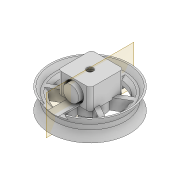
# Autodesk Inventor part: Primary_hinge
Saved by Autodesk Inventor 2022 (Build 260153000, 153)
## iProperties
Created: 2022-07-14
Part Number: Primary_hinge
Material: Generic
Document SubType Name: Modeling
Designer: dell
Density: 1 g/cm^3
Appearance: Default
Mass: 10.1293 g
Surface Area: 99.4908 cm^2
Volume: 10.1293 cm^3
Author: dell
Autodesk Inventor part; units mm, degrees
ref_plane "XZ Plane" through (0, 0, 0) normal (0, 1, 0) x (-1, 0, 0)
ref_plane "XY Plane" through (0, 0, 0) normal (0, 0, 1) x (1, 0, 0)
sketch "Sketch1" plane through (0, 0, 0) normal (0, 0, 1) x (1, 0, 0)
  circle A0 centre (0, 0) radius 4.9
  circle A1 centre (0, 0) radius 6.1
  line L0 (-10.1, -7.1) -> (10.1, -7.1)
  line L1 (10.1, -7.1) -> (10.1, 7.1)
  line L2 (10.1, 7.1) -> (-10.1, 7.1)
  line L3 (-10.1, 7.1) -> (-10.1, -7.1)
  line L4 (-10.1, -7.1) -> (10.1, 7.1) construction
  line L5 (10.1, -7.1) -> (-10.1, 7.1) construction
  dimension "d0" = 9.8
  dimension "d1" = 12.2
  dimension "d3" = 4
  dimension "d4" = 1
  constraints: 12 end point, 2 centre point, 2 coincident, 2 midpoint, 2 parallel, 1 horizontal, 1 perpendicular
  measures "d0" diameter of A0
  measures "d1" diameter of A1
  measures "d3" distance edge to line of A1 L1
  measures "d4" distance edge to line of A1 L2
extrude "Extrusion1" add sketch "Sketch1" along normal blind 18
sketch "Sketch2" plane through (0, 0, 18) normal (0, 0, 1) x (1, 0, 0)
  circle A0 centre (0, 0) radius 4.9 projected
extrude "Extrusion2" add sketch "Sketch2" along normal blind 2
sketch "Sketch3" plane through (0, 0, 0) normal (0, 0, -1) x (-1, 0, 0)
  line L0 (-10.1, -7.1) -> (-10.1, 7.1) projected
  line L1 (10.1, -7.1) -> (-10.1, -7.1) projected
  line L2 (10.1, 7.1) -> (10.1, -7.1) projected
  line L3 (-10.1, 7.1) -> (10.1, 7.1) projected
  circle A0 centre (0, 0) radius 6.1 projected
extrude "Extrusion3" add sketch "Sketch3" along normal blind 3 contours L0 L3 L2 L1 | A0
ref_plane "Work Plane1" through (0, -7.1, 18) normal (-1, 0, 0) x (0, 0, 1)
sketch "Sketch6" plane through (-10.1, 7.1, 18) normal (0, 1, 0) x (1, 0, 0)
  line L0 (5.2, 18) -> (15, 18) projected
  line L1 (16.2, 18) -> (4, 18) projected
  line L2 (20.2, 0) -> (0, 0) projected
  line L3 (0, 21) -> (20.2, 21) projected
  line L4 (16.2, 0) -> (16.2, 18) projected
  line L5 (4, 0) -> (4, 18) projected
  circle A0 centre (10.1, 10) radius 2.05
  line L6 (0, 21) -> (0, 0) projected
  line L7 (20.2, 21) -> (20.2, 0) projected
  point P0 (10.1, 18)
  point P1 (10.1, 18)
  dimension "d49" = 4.1
  dimension "d50" = 10
  constraints: 1 centre point, 1 coincident, 1 midpoint, 1 vertical alignment
  measures "d49" diameter of A0
  measures "d50" distance from line of L2 A0.centre
extrude "Extrusion12" cut sketch "Sketch6" against normal blind 100 contours A0
fillet "Fillet5" radius 2 4 edges at (10.1, 0, 18) (-10.1, 0, 18) (10.1, 0, -3) (-10.1, 0, -3)
sketch "Sketch14" plane through (-8.1, -7.1, -3) normal (0, -1, 0) x (1, 0, 0)
  circle A0 centre (8.1, 11) radius 2.05
  line L0 (8.1, 15.041452) -> (11.6, 13.020726)
  line L1 (11.6, 13.020726) -> (11.6, 8.979274)
  line L2 (11.6, 8.979274) -> (8.1, 6.958548)
  line L3 (8.1, 6.958548) -> (4.6, 8.979274)
  line L4 (4.6, 8.979274) -> (4.6, 13.020726)
  line L5 (4.6, 13.020726) -> (8.1, 15.041452)
  circle A1 centre (8.1, 11) radius 8
  point P0 (8.1, 3)
  dimension "d69" = 7
  dimension "d73" = 16
  constraints: 12 end point, 2 coincident, 1 centre point, 13 other
  measures "d69" distance between parallel lines of L1 L4
  measures "d73" diameter of A1
extrude "Extrusion14" add sketch "Sketch14" along normal blind 5 contours A1
sketch "Sketch15" plane through (0, -12.1, 8) normal (0, -1, 0) x (1, 0, 0)
  line L0 (3.4, -1) -> (4.8, -1)
  line L1 (4.8, -1) -> (4.8, -7.241547)
  line L2 (4.8, -7.241547) -> (3.4, -7.241547)
  line L3 (3.4, -7.241547) -> (3.4, -1)
  line L4 (3.4, -1) -> (4.8, -7.241547) construction
  line L5 (4.8, -1) -> (3.4, -7.241547) construction
  line L6 (0, 16.6) -> (0, -15.6)
  circle A0 centre (0, 0) radius 2.05
  circle A1 centre (0, 0) radius 4.5
  circle A2 centre (0, 0) radius 8
  line L7 (0, 4.041452) -> (3.5, 2.020726)
  line L8 (3.5, 2.020726) -> (3.5, -2.020726)
  line L9 (3.5, -2.020726) -> (0, -4.041452)
  line L10 (0, -4.041452) -> (-3.5, -2.020726)
  line L11 (-3.5, -2.020726) -> (-3.5, 2.020726)
  line L12 (-3.5, 2.020726) -> (0, 4.041452)
  circle A3 centre (0, 0) radius 8
  line L13 (1.4, -7.876547) -> (3.4, -7.876547)
  line L14 (3.4, -7.876547) -> (3.4, -4.876547)
  line L15 (3.4, -4.876547) -> (1.4, -4.876547)
  line L16 (1.4, -4.876547) -> (1.4, -7.876547)
  line L17 (4.8, -6.4) -> (6.8, -6.4)
  line L18 (6.8, -6.4) -> (6.8, -2.4)
  line L19 (6.8, -2.4) -> (4.8, -2.4)
  line L20 (4.8, -2.4) -> (4.8, -6.4)
  line L21 (4.8, 1) -> (3.4, 1)
  line L22 (3.4, 1) -> (3.4, 7.241547)
  line L23 (3.4, 7.241547) -> (4.8, 7.241547)
  line L24 (4.8, 7.241547) -> (4.8, 1)
  line L25 (4.8, 1) -> (3.4, 7.241547) construction
  line L26 (3.4, 1) -> (4.8, 7.241547) construction
  line L27 (4.8, 6.4) -> (6.8, 6.4)
  line L28 (6.8, 6.4) -> (6.8, 3.4)
  line L29 (6.8, 3.4) -> (4.8, 3.4)
  line L30 (4.8, 3.4) -> (4.8, 6.4)
  line L31 (1.4, 8.741547) -> (3.4, 8.741547)
  line L32 (3.4, 8.741547) -> (3.4, 5.741547)
  line L33 (3.4, 5.741547) -> (1.4, 5.741547)
  line L34 (1.4, 5.741547) -> (1.4, 8.741547)
  point P0 (0, -8)
  point P1 (4.1, -4.120773)
  point P2 (4.8, -6.4)
  point P3 (6.8, -4.214262)
  point P4 (4.1, 4.120773)
  point P5 (4.8, 3.4)
  point P6 (6.8, 4.214262)
  point P7 (4.8, 6.4)
  point P8 (1.4, 7.876547)
  point P9 (4.8, 6.4)
  dimension "d74" = 4.1
  dimension "d75" = 1.4
  dimension "d76" = 9
  dimension "d77" = 1
  dimension "d78" = 2
  dimension "d79" = 3
  dimension "d80" = 2
  dimension "d81" = 4
  dimension "d84" = 1.4
  dimension "d85" = 1
  dimension "d86" = 4.1
  dimension "d87" = 2
  dimension "d88" = 3
  dimension "d89" = 2
  dimension "d90" = 3
  dimension "d97" = 1.5
  constraints: 56 end point, 12 parallel, 6 horizontal, 6 perpendicular, 4 midpoint, 4 point on circle, 4 point on line, 1 centre point, 1 coincident, 3 other
  measures "d74" distance from line of L6 point (4.1, -4.121)
  measures "d75" distance between parallel lines of L1 L3
  measures "d76" diameter of A1
  measures "d77" distance from line of A0.centre L0
  measures "d78" distance between parallel lines of L14 L16
  measures "d79" distance between parallel lines of L13 L15
  measures "d80" distance between parallel lines of L1 L18
  measures "d81" distance between parallel lines of L17 L19
  measures "d84" distance between parallel lines of L22 L24
  measures "d85" distance from line of A0.centre L21
  measures "d86" horizontal distance of A0.centre point (4.1, 4.121)
  measures "d87" distance of L28.end L29.end
  measures "d88" distance of L27.end L28.end
  measures "d89" distance of L31.start L31.end
  measures "d90" distance of L33.end L31.start
  measures "d97" distance between parallel lines of L23 L31
extrude "Extrusion15" add sketch "Sketch15" along normal blind 3 contours L33 L34 A2 L22 | L24 A2 L28 L29 | A2 L34 L31 L32 | L27 L28 A2
sketch "Sketch16" plane through (-3.5, -7.1, 5.979274) normal (0, -1, 0) x (1, 0, 0)
  line L0 (3.5, 6.062178) -> (0, 4.041452)
  line L1 (0, 4.041452) -> (0, 0)
  line L2 (0, 0) -> (3.5, -2.020726)
  line L3 (3.5, -2.020726) -> (7, 0)
  line L4 (7, 0) -> (7, 4.041452)
  line L5 (7, 4.041452) -> (3.5, 6.062178)
  circle A0 centre (3.5, 2.020726) radius 2.05
  point P0 (3.5, -5.979274)
extrude "Extrusion16" add sketch "Sketch16" along normal blind 2.4
sketch "Sketch17" plane through (-8.1, -12.1, -3) normal (0, -1, 0) x (1, 0, 0)
  arc A0 (12.9, 17.4) -> (11.5, 18.241547) centre (8.1, 11) ccw
  circle A1 centre (8.1, 11) radius 25
  circle A2 centre (8.1, 11) radius 8
  point P0 (8.1, 3)
  point P1 (9.5, 18.876547)
  point P2 (9.5, 18.876547)
  point P3 (14.9, 15.214262)
  dimension "d94" = 17
  constraints: 2 centre point, 2 coincident, 1 concentric
  measures "d94" radial gap between concentric circles of A0 A1
extrude "Extrusion17" add sketch "Sketch17" against normal blind 2
sketch "Sketch19" plane through (0, 0, 18) normal (0, 0, 1) x (1, 0, 0)
  circle A0 centre (0, 0) radius 4.9 projected
  circle A1 centre (0, 0) radius 6.1 projected
  circle A2 centre (0, 0) radius 4.9 projected
sketch "Sketch18" plane through (-8.1, -7.1, -3) normal (0, -1, 0) x (1, 0, 0)
  circle A0 centre (8.1, 11) radius 25 projected
  arc A1 (-2, 2) -> (0, 0) centre (0, 2) ccw projected
  line L0 (16.2, 0) -> (0, 0) projected
  arc A2 (16.2, 0) -> (18.2, 2) centre (16.2, 2) ccw projected
  line L1 (18.2, 19) -> (18.2, 2) projected
  arc A3 (18.2, 19) -> (16.2, 21) centre (16.2, 19) ccw projected
  line L2 (0, 21) -> (16.2, 21) projected
  arc A4 (0, 21) -> (-2, 19) centre (0, 19) ccw projected
  line L3 (-2, 2) -> (-2, 19) projected
  circle A5 centre (8.1, 11) radius 8 projected
  point P0 (8.1, 3)
extrude "Extrusion18" add sketch "Sketch18" against normal blind 2 contours A0
extrude "Extrusion19" cut sketch "Sketch19" along normal blind 100
thicken "Thicken1" operation add thickness 12 both sides no extend neighbours yes toward (0.9967573, 0, -0.0804666) faces at (7.974058, -8.1, 7.356267)
sketch "Sketch20" plane through (0, -12.1, 8) normal (0, -1, 0) x (1, 0, 0)
  circle A0 centre (0, 0) radius 25 projected
  circle A1 centre (0, 0) radius 22
  point P0 (0, -8)
  dimension "d104" = 3
  constraints: 1 centre point
  measures "d104" radial gap between concentric circles of A0 A1
extrude "Extrusion20" add sketch "Sketch20" along normal blind 3
sketch "Sketch21" plane through (-8.1, -5.1, -3) normal (0, 1, 0) x (1, 0, 0)
  arc A0 (11.44664, -35.774987) -> (4.75336, -35.774987) centre (8.1, -11) ccw
  arc A1 (11.301134, -32.765862) -> (4.898866, -32.765862) centre (8.1, -11) ccw
  circle A2 centre (8.1, -11) radius 2.05
  circle A3 centre (8.1, -11) radius 22
  circle A4 centre (8.1, -11) radius 22
  line L0 (0.1, -31.493902) -> (0.1, -34.685439)
  line L1 (16.1, -31.493902) -> (16.1, -34.685439)
  point P0 (8.1, -3)
  point P1 (11.44664, -33.755219)
  point P2 (4.75336, -33.755219)
  point P3 (16.1, -31.493902)
  point P4 (18.1, -31.712315)
  point P5 (-1.9, -31.712315)
  dimension "d107" = 3
  dimension "d108" = 8
  dimension "d109" = 8
  constraints: 6 point on circle, 4 end point, 2 centre point, 1 coincident, 1 concentric, 1 parallel, 1 vertical
  measures "d107" radial gap between concentric circles of A0 A1
  measures "d108" distance from line of A0.centre L1
  measures "d109" distance from line of A0.centre L0
extrude "Extrusion21" add sketch "Sketch21" along normal blind 3 contours L1 A1 L0 A0
chamfer "Chamfer1" distance 3 distance2 5 1 edges at (-25, -7.1, 8) measured on face at (-24.5, -7.1, 8)
chamfer "Chamfer2" distance 3 distance2 5 1 edges at (-25, -10.1, 8) measured on face at (-24.5, -10.1, 8)
chamfer "Chamfer3" distance 2 distance2 3 1 edges at (0, -2.1, -14) measured on face at (0, -2.1, -14.5)
chamfer "Chamfer4" distance 2 distance2 3 1 edges at (-22, -15.1, 8) measured on face at (-22.5, -15.1, 8)
sketch "Sketch22" plane through (0, -12.1, 8) normal (0, -1, 0) x (1, 0, 0)
  circle A0 centre (0.059205, 0.006086) radius 18.5
  circle A1 centre (0.059205, 0.006086) radius 9.5
  line L0 (-1.5, 18.440263) -> (-1.5, -18.428091)
  line L1 (1.5, -18.437723) -> (1.5, 18.449896)
  line L2 (0, 35) -> (0, -35)
  line L3 (-15.125658, -10.561313) -> (16.803273, 7.872864)
  line L4 (15.311615, 10.475756) -> (-16.634, -7.968053)
  line L5 (16.803273, -7.860691) -> (-15.125658, 10.573486)
  line L6 (-16.634, 7.980226) -> (15.311615, -10.463584)
  arc A2 (8, 21.777052) -> (3.34664, 22.957352) centre (0, 0) ccw
  line L7 (8, 21.777052) -> (8, 20.493902)
  arc A3 (-8, 20.493902) -> (8, 20.493902) centre (0, 0) ccw
  line L8 (-8, 20.493902) -> (-8, 21.777052)
  arc A4 (-3.34664, 22.957352) -> (-8, 21.777052) centre (0, 0) ccw
  line L9 (-3.34664, 22.957352) -> (-3.34664, 10)
  line L10 (-8.1, 10) -> (-3.34664, 10)
  arc A5 (-8.1, 10) -> (-10.1, 8) centre (-8.1, 8) ccw
  line L11 (-10.1, -9) -> (-10.1, 8)
  arc A6 (-10.1, -9) -> (-8.1, -11) centre (-8.1, -9) ccw
  line L12 (8.1, -11) -> (-8.1, -11)
  arc A7 (8.1, -11) -> (10.1, -9) centre (8.1, -9) ccw
  line L13 (10.1, 8) -> (10.1, -9)
  arc A8 (10.1, 8) -> (8.1, 10) centre (8.1, 8) ccw
  line L14 (3.34664, 10) -> (8.1, 10)
  line L15 (3.34664, 10) -> (3.34664, 22.957352)
  point P0 (0, -8)
  point P1 (16.803273, -7.860691)
  point P2 (-1.5, -9.365087)
  point P3 (8.954481, -3.329189)
  point P4 (15.311615, -10.463584)
  point P5 (7.470878, -5.936733)
  point P6 (-7.276867, -6.029811)
  point P7 (-16.634, -7.968053)
  point P8 (-8.793264, -3.441202)
  point P9 (-1.5, 9.377259)
  point P10 (-16.634, 7.980226)
  point P11 (1.5, 9.396193)
  point P12 (-8.793264, 3.453374)
  point P13 (10.1, -3.990555)
  point P14 (10.1, 7.466829)
  point P15 (-15.125658, 10.573486)
  point P16 (16.803273, 7.872864)
  point P17 (8.954481, 3.341362)
  point P18 (1.5, -9.384021)
  point P19 (-10.1, 7.67192)
  point P20 (-1.5, -11)
  point P21 (-10.1, 4.207819)
  point P22 (-10.1, -7.659748)
  point P23 (-3.34664, 18.189876)
  point P24 (-10.088341, 8.21564)
  point P25 (10.064161, 8.376921)
  point P26 (3.34664, 18.211656)
  point P27 (1.5, -11)
  point P28 (10.1, 4.002727)
  point P29 (10.1, -7.454657)
  point P30 (-10.1, -4.195646)
  point P31 (0.177614, 1.738137)
  point P32 (0, 1.840683)
  point P33 (0, 1.635591)
  point P34 (0.177614, -1.725965)
  point P35 (0, -1.623419)
  point P36 (0, -1.82851)
  point P37 (7.470878, 5.948905)
  point P38 (-7.276867, 6.041983)
  dimension "d124" = 37
  dimension "d125" = 19
  dimension "d126" = 1.5
  dimension "d127" = 1.5
  dimension "d130" = 360
  constraints: 12 end point, 4 point on circle, 2 centre point, 1 coincident, 1 vertical, 19 other
  measures "d124" diameter of A0
  measures "d125" diameter of A1
  measures "d126" distance between parallel lines of L2 L1
  measures "d127" distance between parallel lines of L2 L0
extrude "Extrusion22" cut sketch "Sketch22" against normal blind 6 contours A0 L5 L13 L3 | L4 L13 A8 L14 L15 A0 | L13 L5 A1 L3 | A0 L1 L12 A7 L13 L6 | L15 L14 A8 L13 L4 A1 L1 A0 | L13 A7 L12 L1 A1 L6 | A0 L3 L11 A6 L12 L0 | L0 A1 L5 L11 A5 L10 L9 A0 | L4 L2 L5 | L3 L2 L6 | L12 A6 L11 L3 A1 L0 | L9 L10 A5 L11 L5 A0 | A0 L6 L11 L4 | L11 L6 A1 L4
extrude "Extrusion23" cut sketch "Sketch22" against normal blind 8 contours A0 L5 L13 L3 | L4 L13 A8 L14 L15 A0 | A0 L1 L12 A7 L13 L6 | A0 L3 L11 A6 L12 L0 | L3 L2 L6 | L9 L10 A5 L11 L5 A0 | A0 L6 L11 L4
chamfer "Chamfer5" distance 2 angle 45 12 edges at (18.5592, -12.1, 8.0061) (9.3092, -12.1, 24.0276) (9.3092, -12.1, -8.0154) (-9.1908, -12.1, -8.0154) (-18.4408, -12.1, 8.0061) (-9.1908, -12.1, 24.0276) (-18.4408, -5.1, 8.0061) (-9.1908, -5.1, -8.0154) (-9.986, -5.1, 23.5413) (10.1037, -5.1, 23.5418) (18.5592, -5.1, 8.0061) (9.3092, -5.1, -8.0154)
thicken "Thicken2" operation add thickness 2 both sides no extend neighbours yes toward (0.0186792, 0, 0.9998255) faces at (0.373585, -9.1, 27.996511)
body "Solid1"
